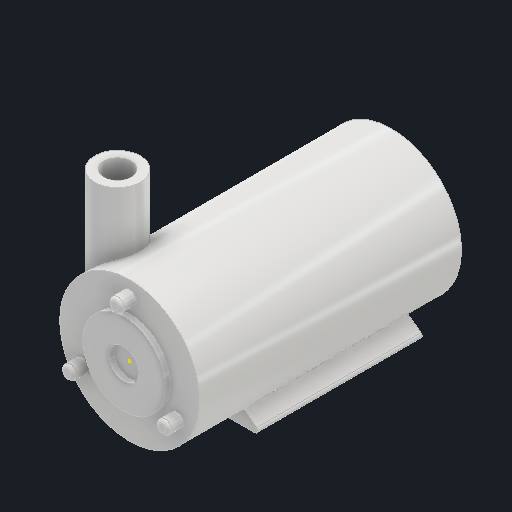
# Autodesk Inventor part: mini_pump
Saved by Autodesk Inventor 2026.2 (Build 302298000, 298)
## iProperties
Created: 2017-08-31
Part Number: mini_pump
Material: ABS Plastic
Document SubType Name: Modeling
Designer: John Nduli
Density: 1.06 g/cm^3
Appearance: Smooth - White
Author: John Nduli
Autodesk Inventor part; units mm, degrees
ref_plane "YZ Plane" through (0, 0, 0) normal (1, 0, 0) x (0, 1, 0)
sketch "Sketch1" plane through (0, 0, 0) normal (0, 1, 0) x (-1, 0, 0)
  circle A0 centre (0, 0) radius 11.5
  dimension "d0" = 23
  constraints: 1 centre point, 1 coincident
  measures "d0" diameter of A0
extrude "Extrusion1" add sketch "Sketch1" along normal blind 43
ref_plane "Work Plane1" through (0, 0, 11.5) normal (0, 0, 1) x (1, 0, 0)
sketch "Sketch2" plane through (0, 0, 11.5) normal (0, 0, 1) x (1, 0, 0)
  circle A0 centre (-7.75, 5.75) radius 3.75
  line L0 (-11.5, 0) -> (11.5, 0) projected
  circle A1 centre (-7.75, 5.75) radius 2.25
  point P0 (0, 0)
  dimension "d3" = 7.5
  dimension "d4" = 5.75
  dimension "d8" = 4.5
  dimension "d41" = 3.75
  constraints: 2 centre point, 1 coincident
  measures "d3" diameter of A0
  measures "d4" distance from line of L0 A0.centre
  measures "d8" diameter of A1
  measures "d41" horizontal distance of L0.start A0.centre
extrude "Extrusion2" add sketch "Sketch2" against normal up to next separate body
sketch "Sketch3" plane through (-7.75, 5.75, 11.5) normal (0, 0, 1) x (1, 0, 0)
  circle A0 centre (0, 0) radius 2.25 projected
  circle A1 centre (0, 0) radius 3.75 projected
  point P0 (7.75, -5.75)
extrude "Extrusion3" add sketch "Sketch3" along normal blind 9 bodies 2
ref_plane "Work Plane2" through (0, 38.5, 0) normal (0, 1, 0) x (1, 0, 0)
sketch "Sketch4" plane through (0, 38.5, 0) normal (0, 1, 0) x (1, 0, 0)
  line L0 (9.0757, 11.5) -> (-9.0757, 11.5)
  circle A0 centre (0, 0) radius 11.5 projected
  line L1 (9.3683, 10.5946) -> (7.1589, 9)
  line L2 (-9.3683, 10.5946) -> (-7.1589, 9)
  circle A1 centre (0, 0) radius 11.5 projected
  line L3 (7.1589, 9) -> (-7.1589, 9)
  arc A2 (-9.0757, 11.5) -> (-9.3683, 10.5946) centre (-9.0757, 11) ccw
  arc A3 (9.3683, 10.5946) -> (9.0757, 11.5) centre (9.0757, 11) ccw
  point P0 (-10.6229, 11.5)
  dimension "d12" = 2.5
  dimension "d13" = 35.818
  dimension "d14" = 0.5
  constraints: 8 end point, 6 point on circle, 5 tangent, 2 centre point, 2 point on line, 1 equal length, 1 equal radius, 1 horizontal, 1 parallel, 2 other
  measures "d12" vertical distance of point (-10.623, 11.5) L2.end
  measures "d13" angle of L0 L2
  measures "d14" radius of A2
extrude "Extrusion4" add sketch "Sketch4" against normal blind 27 contours A3 L1 A0 L0 | A0 L2 A2 L0 bodies 1
sketch "Sketch5" plane through (0, 0, 0) normal (0, -1, 0) x (1, 0, 0)
  circle A0 centre (0, 0) radius 6.75
  circle A1 centre (0, 0) radius 2.5
  dimension "d17" = 13.5
  dimension "d18" = 5
  constraints: 2 centre point, 2 coincident
  measures "d17" diameter of A0
  measures "d18" diameter of A1
extrude "Extrusion5" add sketch "Sketch5" along normal blind 1 bodies 1
sketch "Sketch6" plane through (0, 0, 0) normal (0, -1, 0) x (1, 0, 0)
  point P0 (0, 0)
sketch "Sketch7" plane through (0, 43, 0) normal (0, 1, 0) x (1, 0, 0)
  circle A0 centre (0, 0) radius 2.5 projected
  circle A1 centre (0, 0) radius 10.5
  circle A2 centre (0, 0) radius 11
  dimension "d21" = 22
  dimension "d22" = 21
  constraints: 2 centre point, 2 coincident
  measures "d21" diameter of A2
  measures "d22" diameter of A1
extrude "Extrusion6" cut sketch "Sketch7" against normal blind 2 contours A2 bodies 1
sketch "Sketch8" plane through (0, 43, 0) normal (0, 1, 0) x (1, 0, 0)
  circle A0 centre (0, 5.5) radius 2.75
  circle A1 centre (0, 5.5) radius 2
  circle A2 centre (0, 0) radius 10.5 projected
  dimension "d25" = 4
  dimension "d26" = 5.5
  dimension "d42" = 5.5
  constraints: 2 centre point, 1 coincident, 1 vertical alignment
  measures "d25" diameter of A1
  measures "d26" diameter of A0
  measures "d42" distance of point (0, 0) A0.centre
extrude "Extrusion7" add sketch "Sketch8" along normal blind 1 contours A0 bodies 1
fillet "Fillet1" radius 1 1 edges at (-10.5, 43, 0)
fillet "Fillet2" radius 0.25 2 edges at (-2, 44, -5.5) (-2.75, 44, -5.5)
sketch "Sketch9" plane through (0, 0, 0) normal (0, -1, 0) x (1, 0, 0)
  circle A0 centre (0, 9) radius 1.125
  circle A1 centre (0, 0) radius 11.5 projected
  circle A2 centre (-7.7942, -4.5) radius 1.125
  circle A3 centre (7.7942, -4.5) radius 1.125
  dimension "d32" = 2.25
  dimension "d33" = 9
  dimension "d36" = 360
  constraints: 3 centre point, 1 vertical alignment, 10 other
  measures "d32" diameter of A0
  measures "d33" distance of A1.centre A0.centre
extrude "Extrusion8" add sketch "Sketch9" along normal blind 2.5 contours A0 | A2 | A3 bodies 1
fillet "Fillet3" radius 0.5 3 edges at (6.6692, -2.5, -4.5) (-1.125, -2.5, 9) (-8.9192, -2.5, -4.5)
body "Solid1"
body "Solid2"
